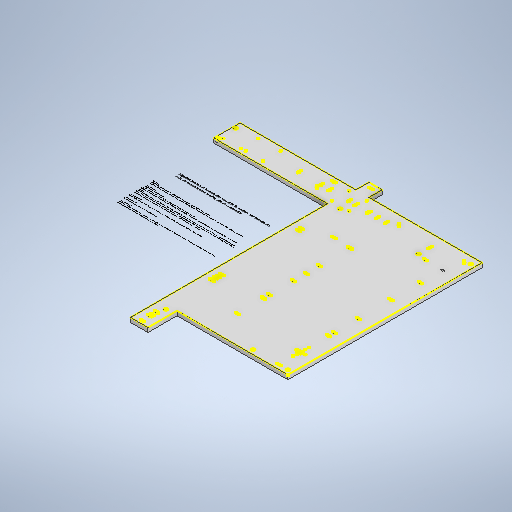
# Autodesk Inventor part: Atlair_PowellandCylindrical_Baseplate_V5
Saved by Autodesk Inventor 2025.2 (Build 292293000, 293)
## iProperties
Created: 2025-04-03
Part Number: Atlair_PowellandCylindrical_Baseplate_V5
Material: Generic
Document SubType Name: Modeling
Designer: Owner
Density: 1 g/cm^3
Appearance: Default
Author: Owner
Autodesk Inventor part; units mm, degrees
(part 1 of 3)
ref_plane "YZ Plane" through (0, 0, 0) normal (1, 0, 0) x (0, 1, 0)
ref_plane "XZ Plane" through (0, 0, 0) normal (0, 1, 0) x (-1, 0, 0)
ref_plane "XY Plane" through (0, 0, 0) normal (0, 0, 1) x (1, 0, 0)
sketch "BoardMounting" plane through (0, 0, 0) normal (0, 1, 0) x (-1, 0, 0)
  line L0 (0, 0) -> (0, -12.7)
  line L1 (0, -12.7) -> (12.7, -12.7)
  circle A0 centre (12.7, -12.7) radius 3.175
  circle A1 centre (12.7, -12.7) radius 5.08
  line L2 (12.7, -12.7) -> (114.3, -12.7)
  line L3 (114.3, -12.7) -> (114.3, -946.404)
  circle A2 centre (114.3, -12.7) radius 3.175
  circle A3 centre (114.3, -12.7) radius 5.08
  line L4 (0, 0) -> (127, 0)
  line L5 (127, 0) -> (127, -964.0878)
  line L6 (127, -964.0878) -> (0, -964.0878)
  line L7 (0, -964.0878) -> (0, 0)
  dimension "d0" = 12.7
  dimension "d1" = 12.7
  dimension "d2" = 6.35
  dimension "d3" = 10.16
  dimension "d4" = 101.6
  dimension "d5" = 933.704
  dimension "d6" = 6.35
  dimension "d7" = 10.16
  dimension "d8" = 127
  constraints: 16 end point, 4 centre point, 4 coincident, 2 horizontal, 2 parallel, 2 perpendicular, 2 vertical
  measures "d0" distance of L0.start L0.end
  measures "d1" distance of L0.end L1.end
  measures "d2" diameter of A0
  measures "d3" diameter of A1
  measures "d4" distance of L2.start L2.end
  measures "d5" distance of L2.end L3.end
  measures "d6" diameter of A2
  measures "d7" diameter of A3
  measures "d8" distance of L5.end L6.end
ref_plane "Work Plane1" through (0, 0, 0) normal (0, 1, 0) x (1, 0, 0)
sketch "Sketch2" plane through (0, 0, 0) normal (0, 1, 0) x (1, 0, 0)
  line L0 (0, 0) -> (-127, 0) projected
  line L1 (0, 0) -> (-38.1, 0)
  line L2 (-38.1, 0) -> (-38.1, 12.7)
  line L3 (-38.1, 12.7) -> (-38.1, 76.2)
  line L4 (-38.1, 76.2) -> (-38.1, 156.845)
  line L5 (-38.1, 156.845) -> (-38.1, 173.736)
  line L6 (-38.1, 173.736) -> (-38.1, 243.84)
  line L7 (-38.1, 243.84) -> (-38.1, 424.2816)
  line L8 (-38.1, 424.2816) -> (-38.1, 489.7374)
  line L9 (-38.1, 489.7374) -> (-38.1, 755.904)
  line L10 (-38.1, 755.904) -> (-38.1, 946.3049)
  line L11 (-38.1, 755.904) -> (-38.1, 794.004)
  line L12 (-38.1, 489.7374) -> (-38.1, 485.9056)
  line L13 (-38.1, 489.7374) -> (-88.9, 489.7374)
  circle A0 centre (-38.1, 12.7) radius 3.175
  line L14 (-38.1, 12.7) -> (-33.096, 12.7)
  line L15 (-38.1, 12.7) -> (-43.104, 12.7)
  circle A1 centre (-43.104, 12.7) radius 1.0125
  circle A2 centre (-33.096, 12.7) radius 1.0125
  circle A3 centre (-38.1, 76.2) radius 3.175
  circle A4 centre (-43.104, 76.2) radius 1.0125
  circle A5 centre (-33.096, 76.2) radius 1.0125
  circle A6 centre (-38.1, 156.845) radius 3.175
  circle A7 centre (-43.104, 156.845) radius 1.0125
  circle A8 centre (-33.096, 156.845) radius 1.0125
  circle A9 centre (-38.1, 173.736) radius 3.175
  circle A10 centre (-43.104, 173.736) radius 1.0125
  circle A11 centre (-33.096, 173.736) radius 1.0125
  circle A12 centre (-38.1, 243.84) radius 3.175
  circle A13 centre (-43.104, 243.84) radius 1.0125
  circle A14 centre (-33.096, 243.84) radius 1.0125
  circle A15 centre (-38.1, 424.2816) radius 3.175
  circle A16 centre (-43.104, 424.2816) radius 1.0125
  circle A17 centre (-33.096, 424.2816) radius 1.0125
  circle A18 centre (-88.9, 489.7374) radius 3.175
  circle A19 centre (-93.904, 489.7374) radius 1.0125
  circle A20 centre (-83.896, 489.7374) radius 1.0125
  circle A21 centre (-38.1, 485.9056) radius 3.175
  circle A22 centre (-43.104, 485.9056) radius 1.0125
  circle A23 centre (-33.096, 485.9056) radius 1.0125
  circle A24 centre (-38.1, 755.904) radius 3.175
  circle A25 centre (-43.104, 755.904) radius 1.016
  circle A26 centre (-33.096, 755.904) radius 1.016
  circle A27 centre (-38.1, 794.004) radius 3.175
  circle A28 centre (-43.104, 794.004) radius 1.016
  circle A29 centre (-33.096, 794.004) radius 1.016
  circle A30 centre (-38.1, 946.3049) radius 3.175
  circle A31 centre (-43.104, 946.3049) radius 1.016
  circle A32 centre (-33.096, 946.3049) radius 1.016
  line L16 (-38.1, 489.7374) -> (-38.1, 527.8374)
  line L17 (-38.1, 527.8374) -> (-266.1666, 527.8374)
  line L18 (-266.1666, 527.8374) -> (-304.2666, 527.8374)
  line L19 (-304.2666, 527.8374) -> (-494.6675, 527.8374)
  line L20 (-37.3622, 527.4138) -> (36.0456, 527.4138) construction
  line L21 (36.0456, 527.4138) -> (36.0456, 504.514) construction
  line L22 (36.0456, 504.514) -> (-37.3622, 504.514) construction
  line L23 (-37.3622, 504.514) -> (-37.3622, 527.4138) construction
  line L24 (-266.1666, 527.8374) -> (-419.1, 527.8374)
  line L25 (-418.2585, 527.0903) -> (-398.4863, 527.0903) construction
  line L26 (-398.4863, 527.0903) -> (-398.4863, 520.8371) construction
  line L27 (-398.4863, 520.8371) -> (-418.2585, 520.8371) construction
  line L28 (-418.2585, 520.8371) -> (-418.2585, 527.0903) construction
  line L29 (-419.1, 527.8374) -> (-419.1, 553.2374)
  line L30 (-419.1, 553.2374) -> (-419.1, 565.9374)
  line L31 (-38.1, 527.8374) -> (-26.0664, 527.8374)
  line L32 (-26.0664, 527.8374) -> (-26.0664, 539.871)
  line L33 (-19.4331, 542.3257) -> (28.6845, 542.3257) construction
  line L34 (28.6845, 542.3257) -> (28.6845, 534.334) construction
  line L35 (28.6845, 534.334) -> (-19.4331, 534.334) construction
  line L36 (-19.4331, 534.334) -> (-19.4331, 542.3257) construction
  circle A33 centre (-26.0664, 539.871) radius 3.175
  circle A34 centre (-29.6048, 543.4093) radius 1.0125
  circle A35 centre (-22.5281, 536.3326) radius 1.0125
  line L37 (-419.1, 527.8374) -> (-419.1, 515.8038)
  line L38 (-419.1, 515.8038) -> (-431.1336, 515.8038)
  circle A36 centre (-431.1336, 515.8038) radius 3.175
  circle A37 centre (-434.6719, 519.3422) radius 1.0125
  circle A38 centre (-427.5952, 512.2655) radius 1.0125
  circle A39 centre (-419.1, 553.2374) radius 3.175
  circle A40 centre (-424.104, 553.2374) radius 1.0125
  circle A41 centre (-414.096, 553.2374) radius 1.0125
  line L39 (-476.1845, 518.6994) -> (-428.0669, 518.6994) construction
  line L40 (-428.0669, 518.6994) -> (-428.0669, 510.7078) construction
  line L41 (-428.0669, 510.7078) -> (-476.1845, 510.7078) construction
  line L42 (-476.1845, 510.7078) -> (-476.1845, 518.6994) construction
  line L43 (-94.3408, 479.1039) -> (-38.4327, 479.1039) construction
  line L44 (-38.4327, 479.1039) -> (-38.4327, 451.7358) construction
  line L45 (-38.4327, 451.7358) -> (-94.3408, 451.7358) construction
  line L46 (-94.3408, 451.7358) -> (-94.3408, 479.1039) construction
  circle A42 centre (-266.1666, 527.8374) radius 3.175
  line L47 (-266.1666, 527.8374) -> (-266.1666, 532.8414)
  line L48 (-266.1666, 527.8374) -> (-266.1666, 522.8334)
  circle A43 centre (-266.1666, 532.8414) radius 1.0125
  circle A44 centre (-266.1666, 522.8334) radius 1.0125
  circle A45 centre (-304.2666, 527.8374) radius 3.175
  circle A46 centre (-304.2666, 532.8414) radius 1.0125
  circle A47 centre (-304.2666, 522.8334) radius 1.0125
  circle A48 centre (-494.6675, 527.8374) radius 3.175
  circle A49 centre (-494.6675, 532.8414) radius 1.0125
  circle A50 centre (-494.6675, 522.8334) radius 1.0125
  line L49 (-419.1, 565.9374) -> (0, 565.9374)
  line L50 (-419.1, 565.9374) -> (-493.6515, 565.9374)
  line L51 (-493.6515, 565.9374) -> (-506.3515, 565.9374)
  line L52 (-494.6675, 527.8374) -> (-494.6675, 489.7374)
  line L53 (-506.3515, 565.9374) -> (-506.3515, 489.7374)
  line L54 (-506.3515, 489.7374) -> (-127, 489.7374)
  line L55 (-127, 0) -> (-127, 964.0878) projected
  line L56 (0, 0) -> (0, 964.0878) projected
  line L57 (-304.2666, 527.8374) -> (-323.3166, 527.8374)
  line L58 (-359.7583, 544.467) -> (-335.55, 544.467) construction
  line L59 (-335.55, 544.467) -> (-335.55, 534.7362) construction
  line L60 (-335.55, 534.7362) -> (-359.7583, 534.7362) construction
  line L61 (-359.7583, 534.7362) -> (-359.7583, 544.467) construction
  line L62 (-323.3166, 527.8374) -> (-323.3166, 404.4684)
  line L63 (-323.3166, 404.4684) -> (-323.3166, 153.0824)
  line L64 (-323.3166, 153.0824) -> (-323.3166, -21.1176)
  line L65 (-323.3166, 489.7374) -> (-285.2166, 489.7374)
  line L66 (-323.3166, 489.7374) -> (-361.4166, 489.7374)
  line L67 (-323.3166, -21.1176) -> (-323.3166, -33.8176)
  line L68 (-323.3166, -33.8176) -> (-361.4166, -33.8176)
  line L69 (-361.4166, -33.8176) -> (-285.2166, -33.8176)
  line L70 (-285.2166, -33.8176) -> (-285.2166, 489.7374)
  line L71 (-285.2166, 489.7374) -> (-361.4166, 489.7374)
  line L72 (-361.4166, 489.7374) -> (-361.4166, -33.8176)
  circle A51 centre (-323.3166, -21.1176) radius 3.175
  circle A52 centre (-328.3206, -21.1176) radius 1.0125
  circle A53 centre (-318.3126, -21.1176) radius 1.0125
  circle A54 centre (-323.3166, 153.0824) radius 3.175
  circle A55 centre (-328.3206, 153.0824) radius 1.0125
  circle A56 centre (-318.3126, 153.0824) radius 1.0125
  circle A57 centre (-323.3166, 404.4684) radius 3.175
  circle A58 centre (-328.3206, 404.4684) radius 1.0125
  circle A59 centre (-318.3126, 404.4684) radius 1.0125
  line L73 (-38.1, 243.84) -> (-38.1, 338.92)
  circle A60 centre (-38.1, 338.92) radius 3.175
  circle A61 centre (-43.104, 338.92) radius 1.0125
  circle A62 centre (-33.096, 338.92) radius 1.0125
  line L74 (-266.1666, 527.8374) -> (-329.6666, 527.8374)
  line L75 (-329.6666, 527.8374) -> (-348.7166, 527.8374)
  circle A63 centre (-329.6666, 522.8334) radius 1.0125
  circle A64 centre (-329.6666, 527.8374) radius 3.175
  circle A65 centre (-329.6666, 532.8414) radius 1.0125
  line L76 (-323.3166, 404.4684) -> (-348.7166, 404.4684)
  line L77 (-348.7166, 404.4684) -> (-348.7166, 379.0684)
  line L78 (-348.7166, 379.0684) -> (-348.7166, 127.6824)
  line L79 (-348.7166, 127.6824) -> (-348.7166, -46.5176)
  line L80 (-348.7166, -46.5176) -> (-348.7166, -59.2176)
  line L81 (-386.8166, -59.2176) -> (-310.6166, -59.2176)
  line L82 (-310.6166, -59.2176) -> (-310.6166, 464.3374)
  line L83 (-386.8166, 464.3374) -> (-386.8166, -59.2176)
  circle A66 centre (-348.7166, -46.5176) radius 3.175
  circle A67 centre (-343.7126, -46.5176) radius 1.0125
  circle A68 centre (-353.7206, -46.5176) radius 1.0125
  circle A69 centre (-348.7166, 127.6824) radius 3.175
  circle A70 centre (-343.7126, 127.6824) radius 1.0125
  circle A71 centre (-353.7206, 127.6824) radius 1.0125
  circle A72 centre (-348.7166, 379.0684) radius 3.175
  circle A73 centre (-343.7126, 379.0684) radius 1.0125
  circle A74 centre (-353.7206, 379.0684) radius 1.0125
  line L84 (-348.7166, 379.0684) -> (-374.1166, 379.0684)
  line L85 (-386.8166, 464.3374) -> (-386.8166, 489.7374)
  line L86 (-310.6166, 464.3374) -> (-310.6166, 489.7374)
  line L87 (-325.5536, 546.4724) -> (-301.3453, 546.4724) construction
  line L88 (-301.3453, 546.4724) -> (-301.3453, 536.7416) construction
  line L89 (-301.3453, 536.7416) -> (-325.5536, 536.7416) construction
  line L90 (-325.5536, 536.7416) -> (-325.5536, 546.4724) construction
  line L91 (-38.1, 485.9056) -> (-38.1, 489.9096)
  circle A75 centre (-38.1, 489.9096) radius 3.175
  circle A76 centre (-43.104, 489.9096) radius 1.0125
  circle A77 centre (-33.096, 489.9096) radius 1.0125
  dimension "d11" = 38.1
  dimension "d12" = 12.7
  dimension "d13" = 63.5
  dimension "d14" = 80.645
  dimension "d15" = 16.891
  dimension "d16" = 70.104
  dimension "d17" = 180.4416
  dimension "d18" = 65.4558
  dimension "d19" = 266.1666
  dimension "d20" = 190.4009
  dimension "d21" = 38.1
  dimension "d22" = 3.8318
  dimension "d23" = 50.8
  dimension "d24" = 6.35
  dimension "d25" = 5.004
  dimension "d26" = 5.004
  dimension "d27" = 2.025
  dimension "d28" = 2.025
  dimension "d29" = 6.35
  dimension "d30" = 5.004
  dimension "d31" = 5.004
  dimension "d32" = 2.025
  dimension "d33" = 2.025
  dimension "d34" = 6.35
  dimension "d35" = 5.004
  dimension "d36" = 5.004
  dimension "d37" = 2.025
  dimension "d38" = 2.025
  dimension "d39" = 6.35
  dimension "d40" = 5.004
  dimension "d41" = 5.004
  dimension "d42" = 2.025
  dimension "d43" = 2.025
  dimension "d44" = 6.35
  dimension "d45" = 5.004
  dimension "d46" = 5.004
  dimension "d47" = 2.025
  dimension "d48" = 2.025
  dimension "d49" = 6.35
  dimension "d50" = 5.004
  dimension "d51" = 5.004
  dimension "d52" = 2.025
  dimension "d53" = 2.025
  dimension "d54" = 6.35
  dimension "d55" = 5.004
  dimension "d56" = 5.004
  dimension "d57" = 2.025
  dimension "d58" = 2.025
  dimension "d59" = 6.35
  dimension "d60" = 5.004
  dimension "d61" = 5.004
  dimension "d62" = 2.025
  dimension "d63" = 2.025
  dimension "d64" = 6.35
  dimension "d65" = 5.004
  dimension "d66" = 5.004
  dimension "d67" = 2.032
  dimension "d68" = 2.032
  dimension "d69" = 6.35
  dimension "d70" = 5.004
  dimension "d71" = 5.004
  dimension "d72" = 2.032
  dimension "d73" = 2.032
  dimension "d74" = 6.35
  constraints: 122 end point, 78 centre point, 64 coincident, 29 point on line, 16 perpendicular, 11 vertical, 7 horizontal, 5 parallel, 9 other
  measures "d11" distance of L0.start L1.end
  measures "d12" distance of L1.end L2.end
  measures "d13" distance of L2.end L3.end
  measures "d14" distance of L3.end L4.end
  measures "d15" distance of L4.end L5.end
  measures "d16" distance of L5.end L6.end
  measures "d17" distance of L6.end L7.end
  measures "d18" distance of L7.end L8.end
  measures "d19" distance of L8.end L9.end
  measures "d20" distance of L9.end L10.end
  measures "d21" distance of L9.end L11.end
  measures "d22" distance of L8.end L12.end
  measures "d23" distance of L8.end L13.end
  measures "d24" diameter of A0
  measures "d25" distance of L14.start L14.end
  measures "d26" distance of L14.start L15.end
  measures "d27" diameter of A1
  measures "d28" diameter of A2
  measures "d29" diameter of A3
  measures "d30" distance of A3.centre point (-33.096, 76.2)
  measures "d31" distance of A3.centre point (-43.104, 76.2)
  measures "d32" diameter of A4
  measures "d33" diameter of A5
  measures "d34" diameter of A6
  measures "d35" distance of A6.centre point (-33.096, 156.845)
  measures "d36" distance of A6.centre point (-43.104, 156.845)
  measures "d37" diameter of A7
  measures "d38" diameter of A8
  measures "d39" diameter of A9
  measures "d40" distance of A9.centre point (-33.096, 173.736)
  measures "d41" distance of A9.centre point (-43.104, 173.736)
  measures "d42" diameter of A10
  measures "d43" diameter of A11
  measures "d44" diameter of A12
  measures "d45" distance of A12.centre point (-33.096, 243.84)
  measures "d46" distance of A12.centre point (-43.104, 243.84)
  measures "d47" diameter of A13
  measures "d48" diameter of A14
  measures "d49" diameter of A15
  measures "d50" distance of A15.centre point (-33.096, 424.282)
  measures "d51" distance of A15.centre point (-43.104, 424.282)
  measures "d52" diameter of A16
  measures "d53" diameter of A17
  measures "d54" diameter of A18
  measures "d55" distance of A18.centre point (-83.896, 489.737)
  measures "d56" distance of A18.centre point (-93.904, 489.737)
  measures "d57" diameter of A19
  measures "d58" diameter of A20
  measures "d59" diameter of A21
  measures "d60" distance of A21.centre point (-33.096, 485.906)
  measures "d61" distance of A21.centre point (-43.104, 485.906)
  measures "d62" diameter of A22
  measures "d63" diameter of A23
  measures "d64" diameter of A24
  measures "d65" distance of A24.centre point (-33.096, 755.904)
  measures "d66" distance of A24.centre point (-43.104, 755.904)
  measures "d67" diameter of A25
  measures "d68" diameter of A26
  measures "d69" diameter of A27
  measures "d70" distance of A27.centre point (-33.096, 794.004)
  measures "d71" distance of A27.centre point (-43.104, 794.004)
  measures "d72" diameter of A28
  measures "d73" diameter of A29
  measures "d74" diameter of A30
extrude "Extrusion4" add sketch "Sketch2" against normal blind 12.7 contours L0 L2 A0 L3 A3 L4 A6 L5 A9 L6 A12 L7 A60 A15 L8 A21 A75 L9 L49 L56 | L0 L55 L17 L9 A75 A21 L8 A15 L7 A60 A12 L6 A9 L5 A6 L4 A3 L3 A0 L2 | L9 L17 L55 L49 | L54 L62 L19 A45 L18 A42 L17 L55 | L55 L17 A42 L18 A45 L19 A64 L29 A39 L30 L49 | L30 A39 L29 L19 A48 L52 A50 L54 L53 L51 L50 | L86 L82 L69 L67 A51 L64 A54 L63 A57 L62 L54 | L62 A57 L76 A58 L77 A72 L84 A74 L72 L54 | L54 L52 A50 A48 L19 A64 L62 | L82 L81 L80 A66 L79 L68 L69 | A21 L8 A75 | A75 L8 A21 | L72 L68 L79 A66 L80 L81 L83 L85 L54 | A57 L63 L62 | L62 L76 A57 | L68 L79 A69 L78 A72 L77 L76 A58 A57 L63 A54 L64 A51 L67 | L84 A74 A72 L78 A69 L79 L68 L72 | A45 L18 L19 | L19 L18 A45 | L63 A57 L76 | A51 L64 L67 | L67 L64 A51 | L84 A74 | A74 L84 | L76 A58 | A58 L76 | L52 A50 | A50 L52 | A54 L64 L63 | L63 L64 A54 | A76 L13 | L13 A76 | A20 L13 | L13 A20 | A1 | A2 | A4 | A5 | A7 | A8 | A10 | A11 | A13 | A14 | A16 | A17 | A19 | A22 | A23 | A34 | A35 | A37 | A38 | A40 | A41 | A43 | A44 | A46 | A47 | A49 | A52 | A53 | A55 | A56 | A59 | A61 | A62 | A63 | A65 | A67 | A68 | A70 | A71 | A73 | A77 picked at (-36.835, 485.9724) picked at (-39.3662, 485.9781)
extrude "ForwardPathDowellPins" cut sketch "Sketch2" against normal blind 4.445 contours L52 A50 | A50 L52 | A76 L13 | L13 A76 | A20 L13 | L13 A20 | A1 | A2 | A4 | A5 | A7 | A8 | A10 | A11 | A13 | A14 | A16 | A17 | A19 | A34 | A35 | A37 | A38 | A40 | A41 | A43 | A44 | A49 | A61 | A62 | A63 | A65 | A77
extrude "ReversePathDowellPins" cut sketch "Sketch2" against normal blind 4.445 contours L84 A74 | A74 L84 | A67 | A68 | A70 | A71 | A73
sketch "CTASLMHoles" plane through (0, 0, 0) normal (0, 1, 0) x (1, 0, 0)
  circle A0 centre (-323.3166, 404.4684) radius 3.175 projected
  circle A1 centre (-328.3206, 404.4684) radius 1.0125 projected
  circle A2 centre (-318.3126, 404.4684) radius 1.0125 projected
  line L0 (-323.3166, 404.4684) -> (-323.3166, 171.2734)
  line L1 (-323.3166, 171.2734) -> (-323.3166, -8.6266)
  circle A3 centre (-323.3166, 171.2734) radius 3.175
  line L2 (-323.3166, 171.2734) -> (-318.3126, 171.2734)
  line L3 (-323.3166, 171.2734) -> (-328.3206, 171.2734)
  circle A4 centre (-318.3126, 171.2734) radius 1.0125
  circle A5 centre (-328.3206, 171.2734) radius 1.0125
  circle A6 centre (-323.3166, -8.6266) radius 3.175
  circle A7 centre (-318.3126, -8.6266) radius 1.0125
  circle A8 centre (-328.3206, -8.6266) radius 1.0125
  line L4 (-323.3166, 404.4684) -> (-348.7166, 404.4684)
  line L5 (-348.7166, 404.4684) -> (-348.7166, 379.0684)
  line L6 (-348.7166, 379.0684) -> (-348.7166, 145.8734)
  line L7 (-348.7166, 145.8734) -> (-348.7166, -34.0266)
  circle A9 centre (-348.7166, 145.8734) radius 3.175
  line L8 (-348.7166, 145.8734) -> (-343.7126, 145.8734)
  line L9 (-348.7166, 145.8734) -> (-353.7206, 145.8734)
  circle A10 centre (-343.7126, 145.8734) radius 1.0125
  circle A11 centre (-353.7206, 145.8734) radius 1.0125
  circle A12 centre (-353.7206, -34.0266) radius 1.0125
  circle A13 centre (-348.7166, -34.0266) radius 3.175
  circle A14 centre (-343.7126, -34.0266) radius 1.0125
  line L10 (-348.7166, 404.4684) -> (-343.7126, 404.4684)
  line L11 (-348.7166, 404.4684) -> (-353.7206, 404.4684)
  circle A15 centre (-348.7166, 379.0684) radius 3.175
  circle A16 centre (-353.7206, 379.0684) radius 1.0125
  circle A17 centre (-343.7126, 379.0684) radius 1.0125
  point P0 (0, 0)
  dimension "d147" = 233.195
  dimension "d148" = 179.9
  dimension "d149" = 6.35
  dimension "d150" = 5.004
  dimension "d151" = 5.004
  dimension "d152" = 2.025
  dimension "d153" = 2.025
  dimension "d154" = 6.35
  dimension "d155" = 5.004
  dimension "d156" = 5.004
  dimension "d157" = 2.025
  dimension "d158" = 2.025
  dimension "d245" = 25.4
  dimension "d246" = 25.4
  dimension "d247" = 233.195
  dimension "d248" = 179.9
  dimension "d249" = 6.35
  dimension "d250" = 5.004
  dimension "d251" = 5.004
  dimension "d252" = 2.025
  dimension "d253" = 2.025
  dimension "d254" = 6.35
  dimension "d255" = 5.004
  dimension "d256" = 5.004
  dimension "d257" = 2.025
  dimension "d258" = 2.025
  dimension "d264" = 6.35
  dimension "d265" = 5.004
  dimension "d266" = 5.004
  dimension "d267" = 2.025
  dimension "d268" = 2.025
  constraints: 24 end point, 16 coincident, 15 centre point, 3 horizontal, 3 perpendicular, 3 point on line, 3 vertical
  measures "d147" distance of L0.start L0.end
  measures "d148" distance of L0.end L1.end
  measures "d149" diameter of A3
  measures "d150" distance of L2.start L2.end
  measures "d151" distance of L2.start L3.end
  measures "d152" diameter of A4
  measures "d153" diameter of A5
  measures "d154" diameter of A6
  measures "d155" distance of A6.centre point (-318.313, -8.627)
  measures "d156" distance of A6.centre point (-328.321, -8.627)
  measures "d157" diameter of A7
  measures "d158" diameter of A8
  measures "d245" distance of L0.start L4.end
  measures "d246" distance of L4.end L5.end
  measures "d247" distance of L6.start L7.start
  measures "d248" distance of L7.start L7.end
  measures "d249" diameter of A9
  measures "d250" distance of L8.start L8.end
  measures "d251" distance of L8.start L9.end
  measures "d252" diameter of A10
  measures "d253" diameter of A11
  measures "d254" diameter of A13
  measures "d255" distance of A13.centre point (-343.713, -34.027)
  measures "d256" distance of A13.centre point (-353.721, -34.027)
  measures "d257" diameter of A14
  measures "d258" diameter of A12
  measures "d264" diameter of A15
  measures "d265" distance of A15.centre point (-343.713, 379.068)
  measures "d266" distance of A15.centre point (-353.721, 379.068)
  measures "d267" diameter of A16
  measures "d268" diameter of A17
sketch "VCSection" plane through (0, 0, 0) normal (0, 1, 0) x (1, 0, 0)
  line L0 (-506.3515, 489.7374) -> (-506.3515, 565.9374) projected
  line L1 (0, 565.9374) -> (0, 0) projected
  line L2 (0, 565.9374) -> (-733.5135, 565.9374)
  circle A0 centre (-494.6675, 527.8374) radius 3.175 projected
  line L3 (-494.6675, 527.8374) -> (-516.8975, 527.8374)
  line L4 (-516.8975, 527.8374) -> (-593.7975, 527.8374)
  line L5 (-593.7975, 527.8374) -> (-596.4935, 527.8374)
  line L6 (-558.6008, 535.3668) -> (-546.0839, 535.3668) construction
  line L7 (-546.0839, 535.3668) -> (-546.0839, 507.3746) construction
  line L8 (-546.0839, 507.3746) -> (-558.6008, 507.3746) construction
  line L9 (-558.6008, 507.3746) -> (-558.6008, 535.3668) construction
  line L10 (-509.4095, 514.9312) -> (-495.072, 514.9312) construction
  line L11 (-495.072, 514.9312) -> (-495.072, 495.8145) construction
  line L12 (-495.072, 495.8145) -> (-509.4095, 495.8145) construction
  line L13 (-509.4095, 495.8145) -> (-509.4095, 514.9312) construction
  line L14 (-598.6701, 547.7163) -> (-575.457, 547.7163) construction
  line L15 (-575.457, 547.7163) -> (-575.457, 536.5649) construction
  line L16 (-575.457, 536.5649) -> (-598.6701, 536.5649) construction
  line L17 (-598.6701, 536.5649) -> (-598.6701, 547.7163) construction
  line L18 (-596.4935, 527.8374) -> (-601.3195, 527.8374)
  line L19 (-604.8621, 516.5149) -> (-593.6053, 516.5149) construction
  line L20 (-593.6053, 516.5149) -> (-593.6053, 497.2176) construction
  line L21 (-593.6053, 497.2176) -> (-604.8621, 497.2176) construction
  line L22 (-604.8621, 497.2176) -> (-604.8621, 516.5149) construction
  line L23 (-645.2026, 600.3199) -> (-327.1795, 600.3199) construction
  line L24 (-327.1795, 600.3199) -> (-327.1795, 572.2467) construction
  line L25 (-327.1795, 572.2467) -> (-645.2026, 572.2467) construction
  line L26 (-645.2026, 572.2467) -> (-645.2026, 600.3199) construction
  line L27 (-601.3195, 527.8374) -> (-639.4195, 527.8374)
  line L28 (-639.4195, 527.8374) -> (-690.2195, 527.8374)
  line L29 (-624.3623, 514.5818) -> (-601.1492, 514.5818) construction
  line L30 (-601.1492, 514.5818) -> (-601.1492, 503.4304) construction
  line L31 (-601.1492, 503.4304) -> (-624.3623, 503.4304) construction
  line L32 (-624.3623, 503.4304) -> (-624.3623, 514.5818) construction
  line L33 (-639.4195, 527.8374) -> (-639.4195, 502.4374)
  line L34 (-639.4195, 527.8374) -> (-639.4195, 553.2374)
  line L35 (-690.2195, 527.8374) -> (-690.2195, 502.4374)
  line L36 (-690.2195, 527.8374) -> (-705.4595, 527.8374)
  line L37 (-705.4595, 527.8374) -> (-705.4595, 565.9374)
  line L38 (-705.4595, 527.8374) -> (-705.4595, 489.7374)
  line L39 (-705.4595, 489.7374) -> (-506.3515, 489.7374)
  point P0 (-506.3515, 565.9374)
  dimension "d160" = 22.23
  dimension "d161" = 76.9
  dimension "d162" = 2.696
  dimension "d163" = 4.826
  dimension "d164" = 38.1
  dimension "d165" = 50.8
  dimension "d166" = 25.4
  dimension "d167" = 25.4
  dimension "d168" = 25.4
  dimension "d169" = 15.24
  constraints: 28 end point, 5 horizontal, 4 point on line, 4 vertical, 2 perpendicular, 12 other
  measures "d160" distance of L3.start L3.end
  measures "d161" distance of L3.end L4.end
  measures "d162" distance of L4.end L5.end
  measures "d163" distance of L5.end L18.end
  measures "d164" distance of L18.end L27.end
  measures "d165" distance of L27.end L28.end
  measures "d166" distance of L27.end L33.end
  measures "d167" distance of L27.end L34.end
  measures "d168" distance of L28.end L35.end
  measures "d169" distance of L28.end L36.end
extrude "VCPlate" add sketch "VCSection" against normal blind 12.7 contours L39 L38 L36 L28 L27 L18 L5 L4 L3 L0 | L3 L4 L5 L18 L27 L28 L36 L37 L2 L0
hole "Hole1" at (-639.4195, 0, -502.4374) at (-690.2195, 0, -502.4374) at (-639.4195, 0, -553.2374) direction (0, -1, 0) diameter 4.9784 end through all thread size "1/4-20 UNC" class "2B" standard "ANSI Unified Screw Threads"
sketch "BaseplateMountingHoles" plane through (0, 0, 0) normal (0, 1, 0) x (1, 0, 0)
  circle A0 centre (-12.7, 12.7) radius 3.175 projected
  circle A1 centre (-12.7, 12.7) radius 5.08 projected
  circle A2 centre (-114.3, 12.7) radius 3.175 projected
  circle A3 centre (-114.3, 12.7) radius 5.08 projected
  line L0 (-12.7, 12.7) -> (-12.7, 546.1)
  line L1 (-12.7, 546.1) -> (-698.5, 546.1)
  line L2 (-698.5, 546.1) -> (-698.5, 495.3)
  line L3 (-698.5, 495.3) -> (-342.9, 495.3)
  line L4 (-342.9, 495.3) -> (-342.9, -12.7)
  line L5 (-342.9, -12.7) -> (-292.1, -12.7)
  line L6 (-292.1, -12.7) -> (-291.0856, 495.3)
  line L7 (-114.3, 12.7) -> (-114.3, 495.3)
  circle A4 centre (-12.7, 546.1) radius 5.08
  circle A5 centre (-12.7, 546.1) radius 3.175
  circle A6 centre (-12.7, 12.7) radius 5.08
  circle A7 centre (-12.7, 12.7) radius 3.175
  circle A8 centre (-114.3, 12.7) radius 5.08
  circle A9 centre (-114.3, 12.7) radius 3.175
  circle A10 centre (-114.3, 495.3) radius 5.08
  circle A11 centre (-114.3, 495.3) radius 3.175
  circle A12 centre (-342.9, 495.3) radius 5.08
  circle A13 centre (-342.9, 495.3) radius 3.175
  circle A14 centre (-291.0856, 495.3) radius 5.08
  circle A15 centre (-291.0856, 495.3) radius 3.175
  circle A16 centre (-292.1, -12.7) radius 5.08
  circle A17 centre (-292.1, -12.7) radius 3.175
  circle A18 centre (-342.9, -12.7) radius 5.08
  circle A19 centre (-342.9, -12.7) radius 3.175
  circle A20 centre (-698.5, 546.1) radius 5.08
  circle A21 centre (-698.5, 546.1) radius 3.175
  circle A22 centre (-698.5, 495.3) radius 5.08
  circle A23 centre (-698.5, 495.3) radius 3.175
  point P0 (0, 0)
  point P1 (-114.3, 12.7)
  dimension "d179" = 533.4
  dimension "d180" = 685.8
  dimension "d181" = 50.8
  dimension "d182" = 355.6
  dimension "d183" = 508
  dimension "d184" = 50.8
  dimension "d185" = 482.6
  dimension "d186" = 10.16
  dimension "d187" = 6.35
  dimension "d188" = 10.16
  dimension "d189" = 6.35
  dimension "d190" = 10.16
  dimension "d191" = 6.35
  dimension "d192" = 10.16
  dimension "d193" = 6.35
  dimension "d194" = 10.16
  dimension "d195" = 6.35
  dimension "d196" = 10.16
  dimension "d197" = 6.35
  dimension "d198" = 10.16
  dimension "d199" = 6.35
  dimension "d200" = 10.16
  dimension "d201" = 6.35
  dimension "d202" = 10.16
  dimension "d203" = 6.35
  dimension "d204" = 10.16
  dimension "d205" = 6.35
  constraints: 20 centre point, 20 coincident, 16 end point, 4 perpendicular, 2 vertical, 1 horizontal, 1 point on line
  measures "d179" distance of L0.start L0.end
  measures "d180" distance of L0.end L1.end
  measures "d181" distance of L1.end L2.end
  measures "d182" distance of L2.end L3.end
  measures "d183" distance of L3.end L4.end
  measures "d184" distance of L4.end L5.end
  measures "d185" distance of L7.start L7.end
  measures "d186" diameter of A4
  measures "d187" diameter of A5
  measures "d188" diameter of A6
  measures "d189" diameter of A7
  measures "d190" diameter of A8
  measures "d191" diameter of A9
  measures "d192" diameter of A10
  measures "d193" diameter of A11
  measures "d194" diameter of A12
  measures "d195" diameter of A13
  measures "d196" diameter of A14
  measures "d197" diameter of A15
  measures "d198" diameter of A16
  measures "d199" diameter of A17
  measures "d200" diameter of A18
  measures "d201" diameter of A19
  measures "d202" diameter of A20
  measures "d203" diameter of A21
  measures "d204" diameter of A22
  measures "d205" diameter of A23
extrude "BaseplateMountingHolesInner" cut sketch "BaseplateMountingHoles" against normal blind 12.7 contours A0 | A2 | A5 L1 L0 | L0 L1 A5 | A21 L2 L1 | L1 L2 A21 | A23 L3 L2 | L2 L3 A23 | A13 L4 L3 | L3 L4 A13 | A19 L5 L4 | L4 L5 A19 | A17 L6 L5 | L5 L6 A17 | A11
extrude "BaseplateMountingHolesOuter" cut sketch "BaseplateMountingHoles" against normal blind 7.62 contours A0 | A1 | A2 | A3 | A4 L1 A5 L0 | L0 A5 L1 A4 | A5 L1 L0 | L0 L1 A5 | A20 L2 A21 L1 | L1 A21 L2 A20 | A21 L2 L1 | L1 L2 A21 | A22 L3 A23 L2 | L2 A23 L3 A22 | A23 L3 L2 | L2 L3 A23 | A12 L4 A13 L3 | L3 A13 L4 A12 | A13 L4 L3 | L3 L4 A13 | A18 L5 A19 L4 | L4 A19 L5 A18 | A19 L5 L4 | L4 L5 A19 | A16 L6 A17 L5 | L5 A17 L6 A16 | A17 L6 L5 | L5 L6 A17 | A10 | A11
extrude "CTASLMElementHolesTop" cut sketch "CTASLMHoles" against normal blind 50.8 contours A9 L8 L6 | L6 L9 A9 | L8 A9 L7 | L7 A9 L9 | A13
extrude "Extrusion10" cut sketch "CTASLMHoles" against normal blind 4.445 contours A10 | A11 | A12 | A14
sketch "ElementHolesBottom" plane through (0, -12.7, 0) normal (0, -1, 0) x (1, 0, 0)
  circle A0 centre (-323.3166, 21.1176) radius 3.175 projected
  circle A1 centre (-323.3166, 8.6266) radius 3.175 projected
  circle A2 centre (-323.3166, -171.2734) radius 3.175 projected
  circle A3 centre (-323.3166, -153.0824) radius 3.175 projected
  circle A4 centre (-323.3166, -404.4684) radius 3.175 projected
  circle A5 centre (-304.2666, -527.8374) radius 3.175 projected
  circle A6 centre (-266.1666, -527.8374) radius 3.175 projected
  circle A7 centre (-431.1336, -515.8038) radius 3.175 projected
  circle A8 centre (-494.6675, -527.8374) radius 3.175 projected
  circle A9 centre (-26.0664, -539.871) radius 3.175 projected
  circle A10 centre (-38.1, -485.9056) radius 3.175 projected
  circle A11 centre (-88.9, -489.7374) radius 3.175 projected
  circle A12 centre (-38.1, -424.2816) radius 3.175 projected
  circle A13 centre (-38.1, -243.84) radius 3.175 projected
  circle A14 centre (-38.1, -173.736) radius 3.175 projected
  circle A15 centre (-38.1, -156.845) radius 3.175 projected
  circle A16 centre (-38.1, -76.2) radius 3.175 projected
  circle A17 centre (-38.1, -12.7) radius 3.175 projected
  circle A18 centre (-419.1, -553.2374) radius 3.175 projected
  circle A19 centre (-38.1, -12.7) radius 5.08
  circle A20 centre (-38.1, -76.2) radius 5.08
  circle A21 centre (-38.1, -156.845) radius 5.08
  circle A22 centre (-38.1, -173.736) radius 5.08
  circle A23 centre (-38.1, -243.84) radius 5.08
  circle A24 centre (-38.1, -424.2816) radius 5.08
  circle A25 centre (-38.1, -485.9056) radius 5.08
  circle A26 centre (-26.0664, -539.871) radius 5.08
  circle A27 centre (-88.9, -489.7374) radius 5.08
  circle A28 centre (-266.1666, -527.8374) radius 5.08
  circle A29 centre (-304.2666, -527.8374) radius 5.08
  circle A30 centre (-323.3166, -404.4684) radius 5.08
  circle A31 centre (-323.3166, -171.2734) radius 5.08
  circle A32 centre (-323.3166, -153.0824) radius 5.08
  circle A33 centre (-323.3166, 21.1176) radius 5.08
  circle A34 centre (-323.3166, 8.6266) radius 5.08
  circle A35 centre (-431.1336, -515.8038) radius 5.08
  circle A36 centre (-419.1, -553.2374) radius 5.08
  circle A37 centre (-494.6675, -527.8374) radius 5.08
  circle A38 centre (-38.1, -338.92) radius 3.175 projected
  circle A39 centre (-38.1, -338.92) radius 5.08
  circle A40 centre (-329.6666, -527.8374) radius 3.175 projected
  circle A41 centre (-348.7166, -127.6824) radius 3.175 projected
  circle A42 centre (-348.7166, -145.8734) radius 3.175 projected
  circle A43 centre (-348.7166, 46.5176) radius 3.175 projected
  circle A44 centre (-348.7166, 34.0266) radius 3.175 projected
  circle A45 centre (-348.7166, -379.0684) radius 3.175 projected
  circle A46 centre (-329.6666, -527.8374) radius 5.08
  circle A47 centre (-348.7166, -379.0684) radius 5.08
  circle A48 centre (-348.7166, -145.8734) radius 5.08
  circle A49 centre (-348.7166, -127.6824) radius 5.08
  circle A50 centre (-348.7166, 34.0266) radius 5.08
  circle A51 centre (-348.7166, 46.5176) radius 5.08
  circle A52 centre (-38.1, -489.9096) radius 3.175 projected
  circle A53 centre (-38.1, -489.9096) radius 5.08
  point P0 (0, 0)
  dimension "d214" = 10.16
  dimension "d215" = 10.16
  dimension "d216" = 10.16
  dimension "d217" = 10.16
  dimension "d218" = 10.16
  dimension "d219" = 10.16
  dimension "d220" = 10.16
  dimension "d221" = 10.16
  dimension "d222" = 10.16
  dimension "d223" = 10.16
  dimension "d224" = 10.16
  dimension "d225" = 10.16
  dimension "d226" = 10.16
  dimension "d227" = 10.16
  dimension "d228" = 10.16
  dimension "d229" = 10.16
  dimension "d230" = 10.16
  dimension "d231" = 10.16
  dimension "d232" = 10.16
  dimension "d239" = 10.16
  dimension "d291" = 10.16
  dimension "d292" = 10.16
  dimension "d293" = 10.16
  dimension "d294" = 10.16
  dimension "d295" = 10.16
  dimension "d296" = 10.16
  dimension "d886" = 10.16
  constraints: 27 centre point, 2 coincident
  measures "d214" diameter of A19
  measures "d215" diameter of A20
  measures "d216" diameter of A21
  measures "d217" diameter of A22
  measures "d218" diameter of A23
  measures "d219" diameter of A24
  measures "d220" diameter of A25
  measures "d221" diameter of A26
  measures "d222" diameter of A27
  measures "d223" diameter of A28
  measures "d224" diameter of A29
  measures "d225" diameter of A30
  measures "d226" diameter of A31
  measures "d227" diameter of A32
  measures "d228" diameter of A33
  measures "d229" diameter of A34
  measures "d230" diameter of A35
  measures "d231" diameter of A36
  measures "d232" diameter of A37
  measures "d239" diameter of A39
  measures "d291" diameter of A46
  measures "d292" diameter of A47
  measures "d293" diameter of A48
  measures "d294" diameter of A49
  measures "d295" diameter of A50
  measures "d296" diameter of A51
  measures "d886" diameter of A53
extrude "Extrusion11" cut sketch "ElementHolesBottom" against normal blind 7.62 contours A6 | A7 | A8 | A9 | A53 A10 A52 | A10 A52 A25 A53 | A53 A25 A52 A10 | A52 A10 | A10 A52 A25 | A25 A52 A53 | A25 A52 | A11 | A12 | A13 | A14 | A15 | A16 | A17 | A18 | A19 | A20 | A21 | A22 | A23 | A24 | A26 | A27 | A28 | A35 | A36 | A37 | A39 | A40 | A41 | A42 | A43 | A44 | A45 | A46 | A47 | A48 | A49 | A50 | A51
sketch "Sketch8" plane through (0, 0, 0) normal (0, 1, 0) x (1, 0, 0)
  line L0 (-665.764, 352.3751) -> (-390.0626, 352.3751) construction
  line L1 (-390.0626, 352.3751) -> (-390.0626, -37.9035) construction
  line L2 (-390.0626, -37.9035) -> (-665.764, -37.9035) construction
  line L3 (-665.764, -37.9035) -> (-665.764, 352.3751) construction
  point P0 (0, 0)
  constraints: 2 other
sketch "CylindricalPath" plane through (0, 0, 0) normal (0, 1, 0) x (1, 0, 0)
  circle A0 centre (-38.1, 12.7) radius 3.175 projected
  line L0 (0, 0) -> (-38.1, 0)
  line L1 (-38.1, 0) -> (-38.1, 12.7)
  line L2 (-38.1, 12.7) -> (-38.1, 88.9)
  line L3 (-38.1, 88.9) -> (-38.1, 106.01)
  line L4 (-38.1, 106.01) -> (-38.1, 176.17)
  line L5 (-38.1, 176.17) -> (-38.1, 214.27)
  line L6 (-38.1, 214.27) -> (-38.1, 252.37)
  line L7 (-38.1, 252.37) -> (-38.1, 345.52)
  line L8 (-38.1, 345.52) -> (-38.1, 523.089)
  line L9 (-38.1, 523.089) -> (-38.1, 561.189)
  line L10 (-38.1, 561.189) -> (-38.1, 661.589)
  line L11 (-38.1, 12.7) -> (-33.096, 12.7)
  line L12 (-38.1, 12.7) -> (-43.104, 12.7)
  circle A1 centre (-33.096, 12.7) radius 1.016
  circle A2 centre (-43.104, 12.7) radius 1.016
  circle A3 centre (-38.1, 12.7) radius 3.175
  circle A4 centre (-38.1, 88.9) radius 3.175
  circle A5 centre (-33.096, 88.9) radius 1.016
  circle A6 centre (-43.104, 88.9) radius 1.016
  line L13 (-38.1, 88.9) -> (-43.104, 88.9)
  line L14 (-38.1, 88.9) -> (-33.096, 88.9)
  circle A7 centre (-38.1, 106.01) radius 3.175
  circle A8 centre (-33.096, 106.01) radius 1.016
  circle A9 centre (-43.104, 106.01) radius 1.016
  line L15 (-38.1, 106.01) -> (-43.104, 106.01)
  line L16 (-38.1, 106.01) -> (-33.096, 106.01)
  circle A10 centre (-38.1, 176.17) radius 3.175
  circle A11 centre (-33.096, 176.17) radius 1.016
  circle A12 centre (-43.104, 176.17) radius 1.016
  line L17 (-38.1, 176.17) -> (-43.104, 176.17)
  line L18 (-38.1, 176.17) -> (-33.096, 176.17)
  circle A13 centre (-38.1, 214.27) radius 3.175
  circle A14 centre (-33.096, 214.27) radius 1.016
  circle A15 centre (-43.104, 214.27) radius 1.016
  line L19 (-38.1, 214.27) -> (-43.104, 214.27)
  line L20 (-38.1, 214.27) -> (-33.096, 214.27)
  circle A16 centre (-38.1, 252.37) radius 3.175
  circle A17 centre (-33.096, 252.37) radius 1.016
  circle A18 centre (-43.104, 252.37) radius 1.016
  line L21 (-38.1, 252.37) -> (-43.104, 252.37)
  line L22 (-38.1, 252.37) -> (-33.096, 252.37)
  circle A19 centre (-38.1, 345.52) radius 3.175
  circle A20 centre (-33.096, 345.52) radius 1.016
  circle A21 centre (-43.104, 345.52) radius 1.016
  line L23 (-38.1, 345.52) -> (-43.104, 345.52)
  line L24 (-38.1, 345.52) -> (-33.096, 345.52)
  circle A22 centre (-38.1, 523.089) radius 3.175
  circle A23 centre (-33.096, 523.089) radius 1.016
  circle A24 centre (-43.104, 523.089) radius 1.016
  line L25 (-38.1, 523.089) -> (-43.104, 523.089)
  line L26 (-38.1, 523.089) -> (-33.096, 523.089)
  circle A25 centre (-38.1, 561.189) radius 3.175
  circle A26 centre (-33.096, 561.189) radius 1.016
  circle A27 centre (-43.104, 561.189) radius 1.016
  line L27 (-38.1, 561.189) -> (-43.104, 561.189)
  line L28 (-38.1, 561.189) -> (-33.096, 561.189)
  circle A28 centre (-38.1, 661.589) radius 3.175
  circle A29 centre (-33.096, 661.589) radius 1.016
  circle A30 centre (-43.104, 661.589) radius 1.016
  line L29 (-38.1, 661.589) -> (-43.104, 661.589)
  line L30 (-38.1, 661.589) -> (-33.096, 661.589)
  line L31 (-63.5, 674.3) -> (-38.1, 674.3)
  line L32 (-38.1, 661.589) -> (-38.1, 674.3)
  line L33 (-38.1, 345.52) -> (-88.9, 345.52)
  circle A31 centre (-88.9, 345.52) radius 3.175
  circle A32 centre (-84.547, 22.1582) radius 1.016
  circle A33 centre (-83.896, 345.52) radius 1.016
  line L34 (-38.1, 345.52) -> (-38.1, 341.6882)
  circle A34 centre (-38.1, 341.6882) radius 3.175
  circle A35 centre (-43.104, 341.6882) radius 1.016
  circle A36 centre (-33.096, 341.6882) radius 1.016
  line L35 (-38.1, 345.52) -> (-38.1, 383.62)
  line L36 (-14.6636, 391.2217) -> (108.4085, 391.2217) construction
  line L37 (108.4085, 391.2217) -> (108.4085, 368.8818) construction
  line L38 (108.4085, 368.8818) -> (-14.6636, 368.8818) construction
  line L39 (-14.6636, 368.8818) -> (-14.6636, 391.2217) construction
  line L40 (-38.1, 345.52) -> (-38.1, 459.82)
  line L41 (-38.1, 459.82) -> (-101.369, 459.82)
  point P0 (0, 0)
  point P1 (-38.1, 341.6882)
  dimension "d297" = 38.1
  dimension "d298" = 12.7
  dimension "d299" = 76.2
  dimension "d300" = 17.11
  dimension "d301" = 70.16
  dimension "d302" = 38.1
  dimension "d303" = 38.1
  dimension "d304" = 93.15
  dimension "d305" = 177.569
  dimension "d306" = 38.1
  dimension "d307" = 100.4
  dimension "d308" = 5.004
  dimension "d309" = 5.004
  dimension "d310" = 2.032
  dimension "d311" = 2.032
  dimension "d312" = 6.35
  dimension "d313" = 5.004
  dimension "d314" = 5.004
  dimension "d315" = 2.032
  dimension "d316" = 2.032
  dimension "d317" = 6.35
  dimension "d318" = 5.004
  dimension "d319" = 5.004
  dimension "d320" = 2.032
  dimension "d321" = 2.032
  dimension "d322" = 6.35
  dimension "d323" = 5.004
  dimension "d324" = 5.004
  dimension "d325" = 2.032
  dimension "d326" = 2.032
  dimension "d327" = 6.35
  dimension "d328" = 5.004
  dimension "d329" = 5.004
  dimension "d330" = 2.032
  dimension "d331" = 2.032
  dimension "d332" = 6.35
  dimension "d333" = 5.004
  dimension "d334" = 5.004
  dimension "d335" = 2.032
  dimension "d336" = 2.032
  dimension "d337" = 6.35
  dimension "d338" = 5.004
  dimension "d339" = 5.004
  dimension "d340" = 2.032
  dimension "d341" = 2.032
  dimension "d342" = 6.35
  dimension "d343" = 5.004
  dimension "d344" = 5.004
  dimension "d345" = 2.032
  dimension "d346" = 2.032
  dimension "d347" = 6.35
  dimension "d348" = 5.004
  dimension "d349" = 5.004
  dimension "d350" = 2.032
  dimension "d351" = 2.032
  dimension "d352" = 6.35
  dimension "d353" = 5.004
  dimension "d354" = 5.004
  dimension "d355" = 2.032
  dimension "d356" = 2.032
  dimension "d357" = 6.35
  dimension "d358" = 50.8
  dimension "d359" = 2.032
  dimension "d360" = 2.032
  constraints: 76 end point, 36 centre point, 30 coincident, 22 horizontal, 9 point on line, 2 vertical, 1 perpendicular, 2 other
  measures "d297" distance of L0.start L1.start
  measures "d298" distance of L1.start L1.end
  measures "d299" distance of L1.end L2.end
  measures "d300" distance of L2.end L3.end
  measures "d301" distance of L3.end L5.start
  measures "d302" distance of L5.start L6.start
  measures "d303" distance of L6.start L6.end
  measures "d304" distance of L6.end L8.start
  measures "d305" distance of L8.start L8.end
  measures "d306" distance of L8.end L9.end
  measures "d307" distance of L9.end L10.end
  measures "d308" distance of L1.end L11.end
  measures "d309" distance of L1.end L12.end
  measures "d310" diameter of A1
  measures "d311" diameter of A2
  measures "d312" diameter of A3
  measures "d313" distance of L13.start L14.end
  measures "d314" distance of L13.start L13.end
  measures "d315" diameter of A5
  measures "d316" diameter of A6
  measures "d317" diameter of A4
  measures "d318" distance of L16.start L16.end
  measures "d319" distance of L16.start L15.end
  measures "d320" diameter of A8
  measures "d321" diameter of A9
  measures "d322" diameter of A7
  measures "d323" distance of L17.start L18.end
  measures "d324" distance of L17.start L17.end
  measures "d325" diameter of A11
  measures "d326" diameter of A12
  measures "d327" diameter of A10
  measures "d328" distance of L19.start L20.end
  measures "d329" distance of L19.start L19.end
  measures "d330" diameter of A14
  measures "d331" diameter of A15
  measures "d332" diameter of A13
  measures "d333" distance of L21.start L22.end
  measures "d334" distance of L21.start L21.end
  measures "d335" diameter of A17
  measures "d336" diameter of A18
  measures "d337" diameter of A16
  measures "d338" distance of L24.start L24.end
  measures "d339" distance of L24.start L23.end
  measures "d340" diameter of A20
  measures "d341" diameter of A21
  measures "d342" diameter of A19
  measures "d343" distance of L26.start L26.end
  measures "d344" distance of L26.start L25.end
  measures "d345" diameter of A23
  measures "d346" diameter of A24
  measures "d347" diameter of A22
  measures "d348" distance of L27.start L28.end
  measures "d349" distance of L27.start L27.end
  measures "d350" diameter of A26
  measures "d351" diameter of A27
  measures "d352" diameter of A25
  measures "d353" distance of L29.start L30.end
  measures "d354" distance of L29.start L29.end
  measures "d355" diameter of A29
  measures "d356" diameter of A30
  measures "d357" diameter of A28
  measures "d358" distance of L24.start L33.end
  measures "d359" diameter of A33
  measures "d360" diameter of A32
sketch "CylindricalPathOption1" plane through (0, 0, 0) normal (0, 1, 0) x (1, 0, 0)
  line L0 (-26.0664, 383.62) -> (-26.0664, 395.6536)
  circle A0 centre (-26.0664, 395.6536) radius 3.175
  circle A1 centre (-29.6048, 399.1919) radius 1.016
  circle A2 centre (-22.5281, 392.1152) radius 1.016
  line L1 (-38.1, 383.62) -> (-26.0664, 383.62)
  line L2 (-38.1, 383.62) -> (-177.569, 383.62)
  circle A3 centre (-177.569, 383.62) radius 3.175
  line L3 (-177.569, 383.62) -> (-215.669, 383.62)
  circle A4 centre (-215.669, 383.62) radius 3.175
  line L4 (-215.669, 383.62) -> (-316.069, 383.62)
  circle A5 centre (-316.069, 383.62) radius 3.175
  line L5 (-215.669, 383.62) -> (-215.669, 281.2623)
  line L6 (-215.669, 383.62) -> (-215.669, 244.84)
  circle A6 centre (-210.629, 244.84) radius 1.016
  circle A7 centre (-220.709, -6.114) radius 1.016
  circle A8 centre (-210.629, -6.114) radius 1.016
  circle A9 centre (-215.669, -6.114) radius 3.175
  line L7 (-215.669, -6.114) -> (-215.669, -219.614)
  circle A10 centre (-210.629, -219.614) radius 1.016
  circle A11 centre (-220.709, -219.614) radius 1.016
  circle A12 centre (-215.669, -219.614) radius 3.175
  line L8 (-215.669, 244.84) -> (-210.629, 244.84)
  line L9 (-215.669, 244.84) -> (-220.709, 244.84)
  circle A13 centre (-220.709, 244.84) radius 1.016
  circle A14 centre (-215.669, 244.84) radius 3.175
  line L10 (-215.669, 244.84) -> (-215.669, -6.114)
  circle A15 centre (-38.1, 345.52) radius 3.175 projected
  circle A16 centre (-88.9, 345.52) radius 3.175 projected
  line L11 (-38.1, 345.52) -> (-38.1, 383.62) projected
  point P0 (0, 0)
  point P1 (-215.669, -219.614)
  point P2 (-220.709, -219.614)
  point P3 (-88.9, 345.52)
  dimension "d396" = 12.0335
  dimension "d397" = 12.0335
  dimension "d398" = 6.35
  dimension "d399" = 2.032
  dimension "d400" = 2.032
  dimension "d401" = 139.469
  dimension "d402" = 6.35
  dimension "d403" = 38.1
  dimension "d404" = 100.4
  dimension "d405" = 138.78
  dimension "d406" = 250.954
  dimension "d407" = 213.5
  dimension "d408" = 5.04
  dimension "d409" = 5.04
  dimension "d410" = 2.032
  dimension "d411" = 2.032
  dimension "d412" = 6.35
  dimension "d413" = 5.04
  dimension "d414" = 5.04
  dimension "d415" = 2.032
  dimension "d416" = 2.032
  dimension "d417" = 6.35
  dimension "d418" = 5.04
  dimension "d419" = 5.04
  dimension "d420" = 2.032
  dimension "d421" = 2.032
  dimension "d422" = 6.35
  constraints: 22 end point, 15 centre point, 12 coincident, 2 horizontal, 2 point on line, 1 perpendicular, 1 vertical
  measures "d396" distance of L2.start L1.end
  measures "d397" distance of L1.end L0.end
  measures "d398" diameter of A0
  measures "d399" diameter of A1
  measures "d400" diameter of A2
  measures "d401" distance of L2.start L2.end
  measures "d402" diameter of A3
  measures "d403" distance of L3.start L3.end
  measures "d404" distance of L5.start L4.end
  measures "d405" distance of L6.start L10.start
  measures "d406" distance of L10.start L10.end
  measures "d407" distance of L10.end L7.end
  measures "d408" distance of L10.start L8.end
  measures "d409" distance of L10.start L9.end
  measures "d410" diameter of A13
  measures "d411" diameter of A6
  measures "d412" diameter of A14
  measures "d413" distance of point (-215.669, -6.114) point (-210.629, -6.114)
  measures "d414" distance of point (-215.669, -6.114) point (-220.709, -6.114)
  measures "d415" diameter of A7
  measures "d416" diameter of A8
  measures "d417" diameter of A9
  measures "d418" distance of point (-215.669, -219.614) point (-210.629, -219.614)
  measures "d419" distance of point (-215.669, -219.614) point (-220.709, -219.614)
  measures "d420" diameter of A11
  measures "d421" diameter of A10
  measures "d422" diameter of A12